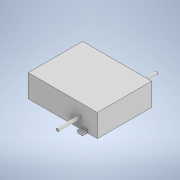
# Autodesk Inventor part: motor
Saved by Autodesk Inventor 2022 (Build 260153000, 153)
## iProperties
Created: 2021-07-05
Part Number: motor
Material: 一般
Document SubType Name: Modeling
Designer: ken
Density: 1 g/cm^3
Appearance: 既定
Author: ken
Autodesk Inventor part; units mm, degrees
ref_plane "YZ Plane" through (0, 0, 0) normal (1, 0, 0) x (0, 1, 0)
ref_plane "XZ Plane" through (0, 0, 0) normal (0, 1, 0) x (-1, 0, 0)
ref_plane "XY Plane" through (0, 0, 0) normal (0, 0, 1) x (1, 0, 0)
sketch "スケッチ1" plane through (0, 0, 0) normal (0, 1, 0) x (-1, 0, 0)
  line L0 (0, 0) -> (70, 0)
  line L1 (70, 0) -> (70, -55)
  line L2 (70, -55) -> (0, -55)
  line L3 (0, -55) -> (0, 0)
  line L4 (60, 0) -> (55, 0)
  line L5 (60, -55) -> (55, -55)
  dimension "d0" = 70
  dimension "d1" = 55
  constraints: 12 end point, 3 horizontal, 2 parallel, 2 point on line, 1 perpendicular
  measures "d0" distance of L1.end L2.end
  measures "d1" distance of L0.end L1.end
extrude "押し出し1" add sketch "スケッチ1" along normal blind 23
sketch "スケッチ2" plane through (0, 0, 0) normal (0, -1, 0) x (1, 0, 0)
  line L0 (-70, 0) -> (0, 0) projected
  line L1 (-10, 0) -> (-15, 0)
  line L2 (-15, 0) -> (-15, 5)
  line L3 (-15, 5) -> (-10, 5)
  line L4 (-10, 5) -> (-10, 0)
  line L5 (0, 0) -> (0, -55) projected
  line L6 (0, -55) -> (-70, -55) projected
  line L7 (-10, -55) -> (-15, -55)
  line L8 (-15, -55) -> (-15, -60)
  line L9 (-15, -60) -> (-10, -60)
  line L10 (-10, -60) -> (-10, -55)
  circle A0 centre (-12.5, 2.5) radius 1.5
  circle A1 centre (-12.5, -57.5) radius 1.5
  dimension "d16" = 5
  dimension "d17" = 5
  dimension "d20" = 10
  dimension "d21" = 5
  dimension "d22" = 5
  dimension "d23" = 10
  dimension "d24" = 3
  dimension "d25" = 3
  dimension "d26" = 2.5
  dimension "d27" = 2.5
  dimension "d28" = 2.5
  dimension "d29" = 2.5
  constraints: 16 end point, 4 parallel, 2 centre point, 2 horizontal, 2 perpendicular, 2 point on line
  measures "d16" distance of L2.end L3.end
  measures "d17" distance of L1.end L2.end
  measures "d20" distance between parallel lines of L5 L4
  measures "d21" distance of L9.end L8.end
  measures "d22" distance of L8.end L7.end
  measures "d23" distance between parallel lines of L5 L10
  measures "d24" diameter of A0
  measures "d25" diameter of A1
  measures "d26" distance from line of A0.centre L4
  measures "d27" distance from line of A0.centre L3
  measures "d28" distance from line of A1.centre L10
  measures "d29" distance from line of A1.centre L9
extrude "押し出し2" add sketch "スケッチ2" against normal blind 3
sketch "スケッチ3" plane through (-70, 23, 0) normal (0, 0, 1) x (1, 0, 0)
  circle A0 centre (52, -13) radius 1.5
  line L0 (70, -23) -> (70, 0) projected
  line L1 (0, -23) -> (55, -23) projected
  dimension "d32" = 3
  dimension "d33" = 18
  dimension "d34" = 10
  constraints: 1 centre point
  measures "d32" diameter of A0
  measures "d33" distance from line of L0 A0.centre
  measures "d34" distance from line of L1 A0.centre
sketch "スケッチ4" plane through (0, 23, -55) normal (0, 0, -1) x (-1, 0, 0)
  circle A0 centre (18, -13) radius 1.5
  line L0 (0, -23) -> (0, 0) projected
  line L1 (15, -23) -> (70, -23) projected
  dimension "d35" = 3
  dimension "d36" = 18
  dimension "d37" = 10
  constraints: 1 centre point
  measures "d35" diameter of A0
  measures "d36" distance from line of L0 A0.centre
  measures "d37" distance from line of L1 A0.centre
extrude "押し出し3" add sketch "スケッチ3" along normal blind 22.5
extrude "押し出し4" add sketch "スケッチ4" along normal blind 22.5
